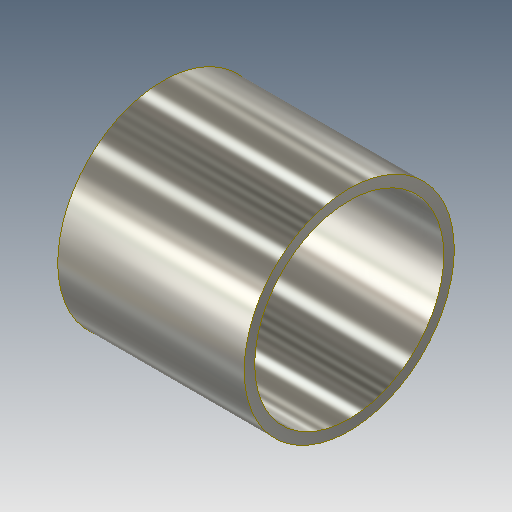
# Autodesk Inventor part: STRUTMOUNT  PART
Saved by Autodesk Inventor 2019 (Build 230136000, 136)
## iProperties
Created: 2023-06-18
Part Number: STRUTMOUNT  PART
Material: Generic
Document SubType Name: Modeling
Designer: Fransic
Density: 1 g/cm^3
Appearance: Silver
Mass: 1.0595 g
Surface Area: 22.3838 cm^2
Volume: 1.0595 cm^3
Author: Fransic
Autodesk Inventor part; units mm, degrees
ref_plane "YZ Plane" through (0, 0, 0) normal (1, 0, 0) x (0, 1, 0)
ref_plane "XZ Plane" through (0, 0, 0) normal (0, 1, 0) x (-1, 0, 0)
ref_plane "XY Plane" through (0, 0, 0) normal (0, 0, 1) x (1, 0, 0)
sketch "Sketch1" plane through (0, 0, 0) normal (1, 0, 0) x (0, 1, 0)
  circle A0 centre (0, 0) radius 10
  dimension "d0" = 20
  constraints: 1 centre point, 1 coincident
  measures "d0" diameter of A0
extrude "Extrusion1" add sketch "Sketch1" along normal blind 17.75
shell "Shell1" thickness 1 removed faces 2 at (0, -1.182, 3.1167) at (17.75, -1.182, 3.1167)
body "Solid1"
